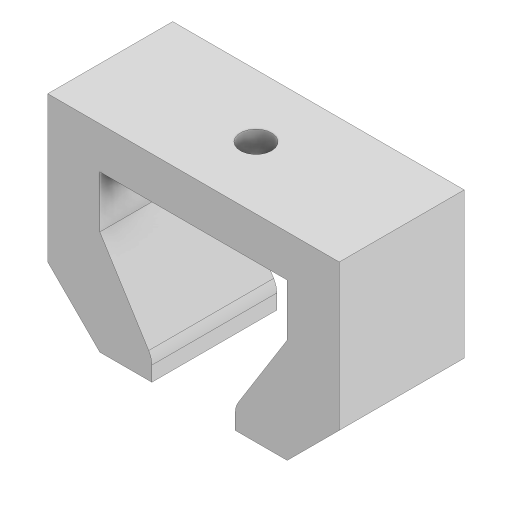
# Autodesk Inventor part: gripper
Saved by Autodesk Inventor 2024 (Build 280153000, 153)
## iProperties
Created: 2023-11-10
Part Number: gripper
Material: 一般
Document SubType Name: Modeling
Designer: moonshot
Density: 1 g/cm^3
Appearance: 既定
Author: moonshot
Autodesk Inventor part; units mm, degrees
ref_plane "YZ Plane" through (0, 0, 0) normal (1, 0, 0) x (0, 1, 0)
ref_plane "XZ Plane" through (0, 0, 0) normal (0, 1, 0) x (-1, 0, 0)
ref_plane "XY Plane" through (0, 0, 0) normal (0, 0, 1) x (1, 0, 0)
sketch "スケッチ1" plane through (0, 0, 0) normal (0, 0, 1) x (1, 0, 0)
  line L0 (-14, 8.973) -> (14, 8.973)
  line L1 (14, 8.973) -> (14, -10.027)
  line L2 (4, -8.027) -> (9, -0.027)
  line L3 (-9, -0.027) -> (-4, -8.027)
  line L4 (-14, -10.027) -> (-14, 8.973)
  line L5 (-4, -8.027) -> (-4, -10.027)
  line L6 (-4, -10.027) -> (-14, -10.027)
  line L7 (4, -8.027) -> (4, -10.027)
  line L8 (4, -10.027) -> (14, -10.027)
  line L9 (0, -13.827) -> (0, 12.773) projected
  line L10 (-9, -0.027) -> (-9, 4.973)
  line L11 (-9, 4.973) -> (9, 4.973)
  line L12 (9, 4.973) -> (9, -0.027)
  point P0 (0, 0)
  dimension "d1" = 8
  dimension "d2" = 18
  dimension "d3" = 10
  dimension "d6" = 2
  dimension "d7" = 5
  dimension "d8" = 4
  dimension "d9" = 15
  constraints: 24 end point, 6 perpendicular, 2 vertical, 1 horizontal, 1 point on line, 4 other
  measures "d1" distance between parallel lines of L7 L5
  measures "d2" distance of L2.end L3.start
  measures "d3" distance of L5.end L4.start
  measures "d6" distance of L3.end L5.end
  measures "d7" distance of L3.start L10.end
  measures "d8" distance between parallel lines of L11 L0
  measures "d9" distance between parallel lines of L6 L11
extrude "押し出し1" add sketch "スケッチ1" along normal mid plane 12
sketch "スケッチ2" plane through (-14, 8.973, 6) normal (0, 1, 0) x (1, 0, 0)
  circle A0 centre (14, 6) radius 1.5
  dimension "d12" = 3
  constraints: 1 centre point, 1 coincident
  measures "d12" diameter of A0
extrude "押し出し2" cut sketch "スケッチ2" against normal through all
fillet "フィレット1" radius 2 2 edges at (-4, -8.027, 0) (4, -8.027, 0)
chamfer "面取り1" distance 5 angle 45 2 edges at (-14, -10.027, 0) (14, -10.027, 0)
